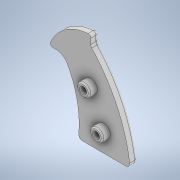
# Autodesk Inventor part: Rukohvat_Desni_4
Saved by Autodesk Inventor 2021 (Build 250183000, 183)
## iProperties
Created: 2022-03-09
Part Number: Rukohvat_Desni_4
Material: Generic
Document SubType Name: Modeling
Designer: Carlos Montoya
Density: 1 g/cm^3
Appearance: Default
Author: Carlos Montoya
Autodesk Inventor part; units mm, degrees
ref_plane "YZ Plane" through (0, 0, 0) normal (1, 0, 0) x (0, 1, 0)
ref_plane "XZ Plane" through (0, 0, 0) normal (0, 1, 0) x (-1, 0, 0)
ref_plane "XY Plane" through (0, 0, 0) normal (0, 0, 1) x (1, 0, 0)
sketch "Sketch1" plane through (0, 0, 0) normal (0, 0, 1) x (1, 0, 0)
  arc A0 (4.1897, 73.9335) -> (-24.7532, 53.8125) centre (6.3147, 40) ccw
  arc A1 (-24.7532, 53.8125) -> (-22.9256, 51) centre (-22.9256, 53) ccw
  line L0 (-22.9256, 51) -> (-20.5538, 51)
  arc A2 (-11.7644, 45.7692) -> (-20.5538, 51) centre (-20.5538, 41) ccw
  arc A3 (-2.9879, 3.2692) -> (-11.7644, 45.7692) centre (-77.6853, 10) ccw
  arc A4 (-2.9879, 3.2692) -> (0, 0) centre (0, 3) ccw
  line L1 (0, 0) -> (33.3057, 0)
  arc A5 (33.3057, 0) -> (36.2787, 3.4018) centre (33.3057, 3) ccw
  arc A6 (36.2787, 3.4018) -> (7.1029, 65.6915) centre (-77.6853, -12) ccw
  arc A7 (6.3147, 67.7183) -> (7.1029, 65.6915) centre (9.3147, 67.7183) ccw
  line L2 (6.3147, 67.7183) -> (6.3147, 71.9374)
  arc A8 (6.3147, 71.9374) -> (4.1897, 73.9335) centre (4.3147, 71.9374) ccw
  circle A9 centre (6.3147, 40) radius 2.75
  circle A10 centre (16.3147, 15) radius 2.75
  constraints: 18 point on circle, 11 centre point, 6 end point
extrude "Extrusion1" add sketch "Sketch1" along normal blind 6
fillet "Fillet1" radius 2 12 edges at (26.457, 36.7791, 0) (6.5187, 66.631, 0) (6.3147, 69.8278, 0) (5.684, 73.3952, 0) (-13.0929, 67.9167, 0) (-24.6027, 51.9103, 0) (-21.7397, 51, 0) (-15.4398, 49.5934, 0) (-4.235, 25.1679, 0) (-2.2145, 0.9761, 0) (16.6529, 0, 0) (35.5646, 1.0258, 0)
chamfer "Chamfer1" distance 2.5 angle 45 1 edges at (3.5647, 40, 0)
chamfer "Chamfer2" distance 2.5 angle 45 1 edges at (13.5647, 15, 0)
sketch "Sketch2" plane through (0, 0, 6) normal (0, 0, 1) x (1, 0, 0)
  circle A0 centre (6.3147, 40) radius 2.75
  circle A1 centre (16.3147, 15) radius 2.75
  circle A2 centre (6.3147, 40) radius 5
  circle A3 centre (16.3147, 15) radius 5
  point P0 (0, 0)
  constraints: 4 centre point
extrude "Extrusion2" add sketch "Sketch2" along normal blind 6
chamfer "Chamfer3" distance 1 angle 45 1 edges at (1.3147, 40, 12)
chamfer "Chamfer4" distance 1 angle 45 1 edges at (11.3147, 15, 12)
body "Solid1"
